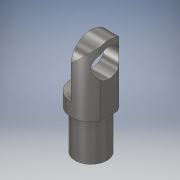
# Autodesk Inventor part: feet type 3 part 2
Saved by Autodesk Inventor 2018 (Build 220112000, 112)
## iProperties
Created: 2018-10-16
Part Number: feet type 3 part 2
Material: Stainless Steel
Document SubType Name: Modeling
Designer: freyja
Density: 8 g/cm^3
Appearance: Semi-Polished
Author: freyja
Autodesk Inventor part; units mm, degrees
ref_plane "YZ Plane" through (0, 0, 0) normal (1, 0, 0) x (0, 1, 0)
ref_plane "XZ Plane" through (0, 0, 0) normal (0, 1, 0) x (-1, 0, 0)
ref_plane "XY Plane" through (0, 0, 0) normal (0, 0, 1) x (1, 0, 0)
sketch "Sketch1" plane through (0, 0, 0) normal (0, 1, 0) x (-1, 0, 0)
  circle A0 centre (0, 0) radius 4.7625
  dimension "d0" = 9.525
  constraints: 1 centre point, 1 coincident
  measures "d0" diameter of A0
extrude "Extrusion1" add sketch "Sketch1" along normal blind 12.7
sketch "Sketch2" plane through (0, 0, 0) normal (0, -1, 0) x (1, 0, 0)
  circle A0 centre (0, 0) radius 2.539
  constraints: 1 centre point, 1 coincident
hole "Hole1" at (0, 0, 0) direction (0, 1, 0) diameter 4.9784 depth 19.05 tip angle 118 thread size "1/4-20 UNC" class "2B" standard "ANSI Unified Screw Threads"
sketch "Sketch3" plane through (0, 12.7, 0) normal (0, 1, 0) x (1, 0, 0)
  circle A0 centre (0, 0) radius 4.7625
  circle A1 centre (0, 0) radius 4.7625 projected
  line L0 (0, -4.7625) -> (0, 4.7625)
  dimension "d10" = 9.525
  constraints: 2 end point, 2 point on circle, 1 centre point, 1 coincident, 1 line through centre, 1 vertical
  measures "d10" diameter of A0
extrude "Extrusion2" add sketch "Sketch3" along normal blind 12.7 contours A0 L0 picked at (1.6786, -1.3984)
sketch "Sketch4" plane through (0, 12.7, -2.4892) normal (-1, 0, 0) x (0, 0, 1)
  line L0 (-2.2733, 0) -> (-2.2733, 12.7) projected
  line L1 (7.2517, 0) -> (7.2517, 12.7) projected
  line L2 (-2.2733, 0) -> (7.2517, 0)
  line L3 (7.2517, 0) -> (7.2517, 12.7)
  line L4 (7.2517, 12.7) -> (-2.2733, 12.7)
  line L5 (-2.2733, 12.7) -> (-2.2733, 0)
  arc A0 (7.2517, 7.9375) -> (-2.2733, 7.9375) centre (2.4892, 7.9375) ccw
  line L6 (7.2517, 12.7) -> (-2.2733, 12.7) projected
  line L7 (-2.2733, 7.9375) -> (-2.2733, 12.7)
  line L8 (-2.2733, 12.7) -> (7.2517, 12.7)
  line L9 (7.2517, 12.7) -> (7.2517, 7.9375)
  point P0 (2.4892, -12.7)
  constraints: 14 end point, 3 equal length, 3 tangent, 2 point on circle, 2 point on line, 1 centre point, 1 horizontal, 1 perpendicular, 1 vertical
extrude "Extrusion3" cut sketch "Sketch4" against normal blind 12.7 contours L0 L4 A0 | L4 L1 A0
sketch "Sketch5" plane through (0, 12.7, -2.4892) normal (-1, 0, 0) x (0, 0, 1)
  arc A0 (7.2517, 7.9375) -> (-2.2733, 7.9375) centre (2.4892, 7.9375) ccw projected
  circle A1 centre (2.4892, 7.9375) radius 2.2013
  point P0 (2.4892, -12.7)
  constraints: 1 centre point, 1 coincident
hole "Hole2" at (0, 20.6375, 0) direction (1, 0, 0) diameter 6.7564 depth 19.05 tip angle 118 clearance for "Flat Head Machine Screw (82)" size "1/4" standard "Ansi Unified Screw Threads"
sketch "Sketch6" plane through (0, 0, 0) normal (0, -1, 0) x (1, 0, 0)
  line L0 (0, 0) -> (4.7909, 0)
  line L1 (5.3024, 5.1468) -> (4.2794, 5.1468)
  line L2 (4.2794, 5.1468) -> (4.2794, -5.1468)
  line L3 (4.2794, -5.1468) -> (5.3024, -5.1468)
  line L4 (5.3024, -5.1468) -> (5.3024, 5.1468)
  line L5 (5.3024, 5.1468) -> (4.2794, -5.1468) construction
  line L6 (4.2794, 5.1468) -> (5.3024, -5.1468) construction
  constraints: 14 end point, 2 horizontal, 2 midpoint, 2 parallel, 1 perpendicular
extrude "Extrusion4" cut sketch "Sketch6" against normal blind 25.4
sketch "Sketch7" plane through (0, 0, 0) normal (0, -1, 0) x (1, 0, 0)
  circle A0 centre (0, 0) radius 4.7625
  circle A1 centre (0, 0) radius 3.81
  dimension "d24" = 9.525
  dimension "d25" = 7.62
  constraints: 2 centre point, 2 coincident
  measures "d24" diameter of A0
  measures "d25" diameter of A1
extrude "Extrusion5" cut sketch "Sketch7" against normal blind 9.525
body "Solid1"
